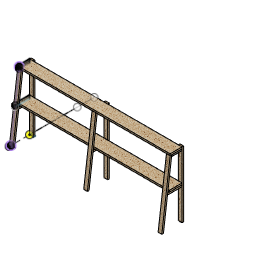
model (Autodesk Fusion 360 design; units mm, degrees)
Autodesk Fusion 360 part; units mm, degrees
note: some values were not read from the file. Set by a fixed rule: which sketch regions a step uses.
sketch "Sketch1" plane through (0, 0, 0) normal (0, 0, 1) x (1, 0, 0)
  line L0 (0, 0) -> (44.45, 0)
  line L1 (44.45, 0) -> (44.45, 19.05)
  line L2 (44.45, 19.05) -> (0, 19.05)
  line L3 (0, 19.05) -> (0, 0)
  line L4 (0, 261.62) -> (44.45, 261.62)
  line L5 (44.45, 261.62) -> (44.45, 242.57)
  line L6 (44.45, 242.57) -> (0, 242.57)
  line L7 (0, 242.57) -> (0, 261.62)
  dimension "d9" = 44.45
  dimension "d10" = 19.05
  dimension "d11" = 44.45
  dimension "d12" = 19.05
  dimension "d13" = 223.52
  constraint horizontal L0
  constraint vertical L1
  constraint horizontal L2
  constraint vertical L3
  constraint coincident L0.start L3.end
  constraint horizontal L4
  constraint vertical L5
  constraint horizontal L6
  constraint vertical L7
  measures "d9" distance of L0.start L0.end
  measures "d10" distance of L0.start L2.end
  measures "d11" distance of L4.start L4.end
  measures "d12" distance of L4.start L6.end
  measures "d13" distance of L2 L6
sketch "Sketch2" plane through (0, 0, 0) normal (1, 0, 0) x (0, 1, 0)
  line L0 (19.05, 0) -> (119.2059, 768.2079)
  line L1 (19.05, 0) -> (814.386, 0) construction
  line L2 (280.67, 0) -> (1017.5859, 0) construction
  point P0 (19.05, 0)
  dimension "d29" = 82.572
  dimension "d30" = 774.7094
  dimension "d33" = 280.67
  constraint horizontal L1
  constraint horizontal L2
  constraint coincident L1 L2.start
  constraint coincident P0 L0.start
  measures "d29" angle of L0 L1
  measures "d30" distance of P0 L0.end
  measures "d33" distance of origin L2.start
sketch "Sketch3" plane through (0, 0, 0) normal (1, 0, 0) x (0, 1, 0)
  line L0 (242.57, 787.4) -> (99.06, 787.4)
  line L1 (99.06, 787.4) -> (99.06, 768.35)
  line L2 (99.06, 768.35) -> (242.57, 768.35)
  line L3 (242.57, 768.35) -> (242.57, 787.4)
  line L4 (242.57, 412.75) -> (90.17, 412.75)
  line L5 (90.17, 412.75) -> (90.17, 393.7)
  line L6 (90.17, 393.7) -> (242.57, 393.7)
  line L7 (242.57, 393.7) -> (242.57, 412.75)
  line L8 (90.17, 393.7) -> (70.379, 393.7)
  line L9 (19.05, 0) -> (119.2059, 768.2079)
  line L10 (242.57, 393.7) -> (242.57, 374.65)
  line L11 (242.57, 374.65) -> (67.9131, 374.7863)
  line L12 (70.379, 393.7) -> (67.9131, 374.7863)
  line L13 (242.57, 768.35) -> (119.2244, 768.35)
  line L14 (242.57, 768.35) -> (242.57, 749.3)
  line L15 (242.57, 749.3) -> (116.7407, 749.3)
  line L16 (116.7407, 749.3) -> (119.2244, 768.35)
  point P0 (242.57, 0)
  dimension "d66" = 787.4
  dimension "d67" = 143.51
  dimension "d68" = 19.05
  dimension "d69" = 152.4
  dimension "d70" = 19.05
  dimension "d71" = 355.6
  dimension "d72" = 787.4
  dimension "d75" = 19.05
  dimension "d86" = 19.05
  constraint horizontal L0
  constraint vertical L1
  constraint horizontal L2
  constraint vertical L3
  constraint horizontal L4
  constraint vertical L5
  constraint horizontal L6
  constraint vertical L7
  constraint perpendicular L5 L8
  constraint coincident L8.end L9
  constraint coincident L9 L11.end
  constraint horizontal L13
  constraint coincident L9 L13.end
  constraint perpendicular L13 L14
  constraint coincident L9 L15.end
  constraint perpendicular L3 L15
  constraint collinear L10 L14
  measures "d66" distance of L0.start P0
  measures "d67" distance of L0.start L0.end
  measures "d68" distance of L0.start L2.end
  measures "d69" distance of L4.start L4.end
  measures "d70" distance of L4.start L6.end
  measures "d71" distance of L2 L4
  measures "d72" distance of P0 L0
  measures "d75" distance of L6.end L10.end
  measures "d86" distance of L2.end L14.end
extrude "Extrude3" add sketch "Sketch1" along normal blind 787.4 contours L4 L5 L6 L7 makes body 1
extrude "Extrude4" add sketch "Sketch3" along normal blind 1828.8 separate body contours L0 L1 L2 L3 L13 | L4 L5 L6 L7 makes body 2 at (609.6, 194.7333, 787.4) makes body 3 at (609.6, 140.97, 393.7)
extrude "Extrude5" add sketch "Sketch3" along normal blind 44.45 separate body contours L2 L9 L13 L14 L15 L16 | L6 L8 L9 L10 L11 L12 makes body 4 at (29.6333, 126.1321, 374.7408) makes body 5 at (14.8167, 200.6269, 749.3)
sweep "Sweep4" add profiles "Sketch1" path "Sketch2" along L0 section 1 contours L0 L1 L2 L3 separate body makes body 6
copy_body "Body->Comp1" bodies 6 removing the originals makes body 7 in component "Leg Assembly"
copy_body "CutPasteBodies1" bodies 5 removing the originals makes body 8 in component "Leg Assembly"
copy_body "CutPasteBodies2" bodies 4 removing the originals makes body 9 in component "Leg Assembly"
copy_body "CutPasteBodies3" bodies 1 removing the originals makes body 10 in component "Leg Assembly"
pattern_linear "먁29" [suppressed]
component "Leg Assembly" placed x (1, 0, 0) y (0, 1, 0) z (0, 0, 1) at (0, 0, 0)
component "Leg Assembly" placed x (1, 0, 0) y (0, 1, 0) z (0, 0, 1) at (892.175, 0, 0)
component "Leg Assembly" placed x (1, 0, 0) y (0, 1, 0) z (0, 0, 1) at (1784.35, 0, 0)
equation "TableLength = 72 in"
equation "LegWoodDepth = 0.75 in"
equation "LegWoodWidth = 1.75 in"
equation "TableTopWidth = 5.65 in"
equation "TableShelfWidth = 6 in"
equation "TableBottomWidth = 9.55 in"
equation "TableShelfHeight = 14 in"
equation "TableSurfaceHeight = 0.75 in"
equation "d9 = LegWoodWidth"
equation "d10 = LegWoodDepth"
equation "d11 = LegWoodWidth"
equation "d12 = LegWoodDepth"
equation "d13 = TableBottomWidth - LegWoodDepth"
equation "TableHeight = 31 in"
equation "LegAngle = ( tan(( ( TableBottomWidth - ( TableTopWidth ) ) / ( TableHeight - TableSurfaceHeight ) ) * 1 rad) ) * 1 rad"
equation "LegLength = ( ( ( ( TableBottomWidth - TableTopWidth ) / 1 in ) ^ 2 + ( ( TableHeight - TableSurfaceHeight ) / 1 in ) ^ 2 ) ^ ( 1 / 2 ) ) * 1 in"
equation "d29 = 90 deg - LegAngle"
equation "d30 = LegLength"
equation "d33 = TableBottomWidth + LegWoodDepth * 2"
equation "d58 = TableHeight"
equation "d66 = TableHeight"
equation "d67 = TableTopWidth"
equation "d68 = TableSurfaceHeight"
equation "d69 = TableShelfWidth"
equation "d70 = TableSurfaceHeight"
equation "d71 = TableShelfHeight"
equation "d72 = TableHeight"
equation "d73 = TableLength"
equation "d75 = LegWoodDepth"
equation "d77 = LegWoodWidth"
equation "LegAngleDeg = LegAngle"
equation "d86 = LegWoodDepth"
equation "d89 = TableLength - LegWoodWidth"
named bodies: "Top Shelf", "Bottom Shelf"
